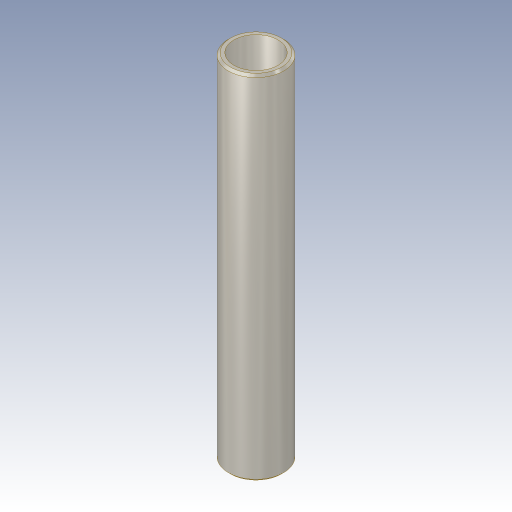
# Autodesk Inventor part: BT005_huenin20_23
Saved by Autodesk Inventor 2023.3 (Build 273359000, 359)
## iProperties
Company: HTBLA Kaindorf
RuleStatus: InUse
Created: 2023-08-29
Part Number: BT005_huenin20_23
Project: Fiberprinter-Hotend
Material: Titan
Description: Mountingconectors
Document SubType Name: Modeling
Designer: huenin20
Density: 4.51 g/cm^3
Appearance: Titan
Mass: 0.127172 g
Surface Area: 2.28783 cm^2
Volume: 0.0281979 cm^3
AfterDocNew0: iProperties-Editor_aufrufen
Author: nicob
Keywords: 2023
Autodesk Inventor part; units mm, degrees
ref_plane "YZ Plane" through (0, 0, 0) normal (1, 0, 0) x (0, 1, 0)
ref_plane "XZ Plane" through (0, 0, 0) normal (0, 1, 0) x (-1, 0, 0)
ref_plane "XY Plane" through (0, 0, 0) normal (0, 0, 1) x (1, 0, 0)
sketch "Skizze3" plane through (0, 0, 0) normal (1, 0, 0) x (0, 1, 0)
  line L0 (0, 0) -> (0, 8.4101)
  line L1 (-1, 0) -> (-1, 16)
  line L2 (-1, 16) -> (-1.25, 16)
  line L3 (-1.25, 16) -> (-1.25, 0)
  line L4 (-1.25, 0) -> (-1, 0)
  dimension "d4" = 2.5
  dimension "d5" = 16
  dimension "d6" = 2
  constraints: 10 end point, 3 perpendicular, 2 vertical, 1 horizontal alignment
  measures "d4" diameter of L3 L0
  measures "d5" distance of L2.end L3.end
  measures "d6" diameter of L1 L0
revolve "Umdrehung1" add sketch "Skizze3" angle 360 about axis through (0, 0, 0) along (0, 0, 1)
chamfer "Fase1" distance 0.1 angle 45 2 edges at (0, 1.25, 16) (0, 1.25, 0)
